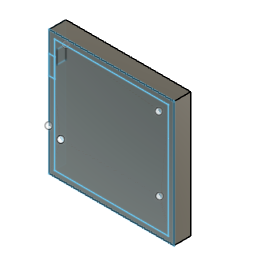
Enclosure Version final (Autodesk Fusion 360 design; units mm, degrees)
Autodesk Fusion 360 part; units mm, degrees
sketch "Sketch1" plane through (0, 0, 0) normal (0, 1, 0) x (1, 0, 0)
  line L0 (0, -75) -> (112, -75)
  line L1 (112, -75) -> (112, 37)
  line L2 (112, 37) -> (0, 37)
  line L3 (0, 37) -> (0, -75)
  line L4 (5, -70) -> (107, -70)
  line L5 (107, -70) -> (107, 32)
  line L6 (107, 32) -> (5, 32)
  line L7 (5, 32) -> (5, -70)
  circle A0 centre (10.441, -30) radius 1.25
  circle A1 centre (98.74, -60.5836) radius 1.25
  circle A2 centre (99.436, 4.9952) radius 1.25
  dimension "d1" = 112
  dimension "d2" = 112
  dimension "d3" = 102
  dimension "d4" = 102
  dimension "d6" = 2.5
  dimension "d8" = 2.5
  dimension "d10" = 2.5
  constraint horizontal L0
  constraint vertical L1
  constraint horizontal L2
  constraint vertical L3
  constraint horizontal L4
  constraint vertical L5
  constraint horizontal L6
  constraint vertical L7
  measures "d1" distance of L0.start L0.end
  measures "d2" distance of L0.end L1.end
  measures "d3" distance of L4.start L4.end
  measures "d4" distance of L4.end L5.end
  measures "d6" diameter of A0
  measures "d8" diameter of A1
  measures "d10" diameter of A2
sketch "Sketch2" plane through (0, 0, 0) normal (0, 1, 0) x (1, 0, 0)
  line L0 (112.6206, 112.7985) -> (10.6206, 112.7985)
  circle A0 centre (16.0616, 86.0944) radius 1.25
  line L1 (10.6206, 10.7985) -> (112.6206, 10.7985)
  line L2 (117.6206, 117.7985) -> (5.6206, 117.7985)
  circle A1 centre (104.7343, 85.7937) radius 1.25
  line L3 (117.6206, 5.7985) -> (117.6206, 117.7985)
  line L4 (5.6206, 117.7985) -> (5.6206, 5.7985)
  line L5 (5.6206, 5.7985) -> (117.6206, 5.7985)
  line L6 (10.6206, 112.7985) -> (10.6206, 10.7985)
  line L7 (112.6206, 10.7985) -> (112.6206, 112.7985)
  circle A2 centre (104.0383, 20.2149) radius 1.25
  circle A3 centre (16.0616, 86.0944) radius 1.75
  line L8 (10.6206, 41.7936) -> (5.6206, 41.7936)
  line L9 (5.6206, 41.7936) -> (5.6206, 24.5486)
  line L10 (5.6206, 24.5486) -> (10.6206, 24.5486)
  line L11 (10.6206, 24.5486) -> (10.6206, 41.7936)
  point P0 (5.2983, 80.7985)
  dimension "d11" = 112
  dimension "d12" = 112
  dimension "d13" = 102
  dimension "d14" = 102
  dimension "d15" = 2.5
  dimension "d16" = 2.5
  dimension "d17" = 2.5
  dimension "d22" = 3.5
  constraint horizontal L5
  constraint vertical L3
  constraint horizontal L2
  constraint vertical L4
  constraint horizontal L1
  constraint vertical L7
  constraint horizontal L0
  constraint vertical L6
  constraint concentric A0 A3
  constraint horizontal L8
  constraint vertical L9
  constraint horizontal L10
  constraint vertical L11
  constraint coincident L4 L9.end
  constraint coincident L6 L8.start
  measures "d11" distance of L4.end L3.start
  measures "d12" distance of L2.start L3.start
  measures "d13" distance of L1.end L1.start
  measures "d14" distance of L1.end L0.start
  measures "d15" diameter of A0
  measures "d16" diameter of A2
  measures "d17" diameter of A1
  measures "d22" diameter of A3
extrude "Extrude1" add sketch "Sketch2" along normal blind 15 contours L0 L1 L2 L3 L4 L5 L6 L7 L8 L10 | L4 L6 L8 L9 L10 L11
extrude "Extrude2" add sketch "Sketch2" along normal blind 5 contours L0 L1 L6 L7 L11 | A3
sketch "Sketch3" plane through (0, 0, 0) normal (0, 1, 0) x (1, 0, 0)
other "Base Mesh Feature3"
other "Modify1"
other "Modify2"
sketch "Sketch4" plane through (5.6206, 0, 0) normal (-1, 0, 0) x (0, -1, 0)
  line L0 (0, -117.7985) -> (0, -5.7985)
  line L1 (0, -5.7985) -> (-15, -5.7985)
  line L2 (-15, -5.7985) -> (-15, -117.7985)
  line L3 (-15, -117.7985) -> (0, -117.7985)
  line L4 (-15, -24.8598) -> (-7, -24.8598)
  line L5 (-7, -24.8598) -> (-7, -36.8598)
  line L6 (-7, -36.8598) -> (-15, -36.8598)
  line L7 (-15, -36.8598) -> (-15, -24.8598)
  dimension "d29" = 12
  dimension "d33" = 8
  constraint horizontal L4
  constraint vertical L5
  constraint horizontal L6
  constraint vertical L7
  constraint coincident L2 L4.start
  measures "d29" distance of L4.start L6.end
  measures "d33" distance of L4.start L4.end
other "Modify3"
extrude "Extrude6" [suppressed]
extrude "Extrude5" [suppressed]
extrude "Extrude4" [suppressed]
extrude "Extrude3" [suppressed]
